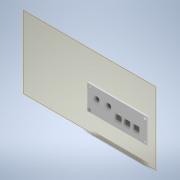
# Autodesk Inventor part: InterfacePlate
Saved by Autodesk Inventor 2022.2 (Build 262287000, 287)
## iProperties
Created: 2022-01-15
Part Number: InterfacePlate
Material: Generic
Document SubType Name: Modeling
Designer: siwat
Density: 1 g/cm^3
Appearance: Default
Author: siwat
Autodesk Inventor part; units mm, degrees
ref_plane "YZ Plane" through (0, 0, 0) normal (1, 0, 0) x (0, 1, 0)
ref_plane "XZ Plane" through (0, 0, 0) normal (0, 1, 0) x (-1, 0, 0)
ref_plane "XY Plane" through (0, 0, 0) normal (0, 0, 1) x (1, 0, 0)
ref_plane "Work Plane1" through (0, 0, 0) normal (0, 0, 1) x (1, 0, 0)
sketch "Sketch1" plane through (0, 0, 0) normal (0, 0, 1) x (1, 0, 0)
  line L0 (67.7271, 45.3897) -> (135.6749, 45.3897)
  line L1 (135.6749, 45.3897) -> (135.6749, 17.2701)
  line L2 (135.6749, 17.2701) -> (67.7271, 17.2701)
  line L3 (67.7271, 17.2701) -> (67.7271, 45.3897)
  circle A0 centre (70.3236, 42.7621) radius 1.5
  circle A1 centre (70.2655, 19.7679) radius 1.5
  circle A2 centre (132.8977, 19.6632) radius 1.5
  circle A3 centre (132.9442, 42.6673) radius 1.5
  point P0 (0, 0)
  dimension "d0" = 3
  dimension "d1" = 3
  dimension "d2" = 3
  dimension "d3" = 3
  constraints: 8 end point, 4 centre point, 2 parallel, 1 horizontal, 1 perpendicular
  measures "d0" diameter of A0
  measures "d1" diameter of A1
  measures "d2" diameter of A2
  measures "d3" diameter of A3
extrude "Extrusion1" add sketch "Sketch1" along normal blind 2
sketch "Sketch2" plane through (0, 0, 0) normal (0, 0, -1) x (-1, 0, 0)
  line L0 (-130.1897, 21.9638) -> (-72.4709, 21.9638)
  line L1 (-72.4709, 21.9638) -> (-72.4709, 40.332)
  line L2 (-72.4709, 40.332) -> (-130.1897, 40.332)
  line L3 (-130.1897, 40.332) -> (-130.1897, 21.9638)
  point P0 (0, 0)
  constraints: 8 end point, 2 parallel, 1 horizontal, 1 perpendicular
extrude "Extrusion2" add sketch "Sketch2" along normal blind 3
sketch "Sketch3" plane through (0, 0, -3) normal (0, 0, -1) x (-1, 0, 0)
  circle A0 centre (-123.1484, 27.6797) radius 2
  line L0 (-121.6186, 32.121) -> (-111.2555, 32.121)
  circle A1 centre (-113.1484, 27.6797) radius 2
  circle A2 centre (-103.1484, 27.6797) radius 2
  circle A3 centre (-91.5974, 33.7589) radius 2.65
  circle A4 centre (-78.3445, 33.7589) radius 2.65
  point P0 (0, 0)
  dimension "d8" = 4
  dimension "d11" = 10
  dimension "d16" = 5.3
  dimension "d17" = 5.3
  constraints: 5 centre point, 2 end point, 2 horizontal, 4 other
  measures "d8" diameter of A0
  measures "d11" distance of A0.centre A1.centre
  measures "d16" diameter of A3
  measures "d17" diameter of A4
extrude "Extrusion3" cut sketch "Sketch3" against normal up to surface (5 mm away)
sketch "Sketch5" plane through (0, 0, 2) normal (0, 0, 1) x (1, 0, 0)
  circle A0 centre (78.3445, 33.7589) radius 2.65 projected
  circle A1 centre (78.3445, 33.7589) radius 3.5
  circle A2 centre (91.5974, 33.7589) radius 2.65 projected
  circle A3 centre (91.5974, 33.7589) radius 3.5
  point P0 (0, 0)
  dimension "d22" = 7
  dimension "d23" = 7
  constraints: 2 centre point, 2 coincident
  measures "d22" diameter of A1
  measures "d23" diameter of A3
extrude "Extrusion5" cut sketch "Sketch5" against normal blind 0.5
sketch "Sketch6" plane through (0, 0, 2) normal (0, 0, 1) x (1, 0, 0)
  line L0 (99.7984, 31.0297) -> (106.4984, 31.0297)
  line L1 (106.4984, 31.0297) -> (106.4984, 24.3297)
  line L2 (106.4984, 24.3297) -> (99.7984, 24.3297)
  line L3 (99.7984, 24.3297) -> (99.7984, 31.0297)
  circle A0 centre (103.1484, 27.6797) radius 2 projected
  line L4 (109.7984, 31.0297) -> (116.4984, 31.0297)
  line L5 (116.4984, 31.0297) -> (116.4984, 24.3297)
  line L6 (116.4984, 24.3297) -> (109.7984, 24.3297)
  line L7 (109.7984, 24.3297) -> (109.7984, 31.0297)
  line L8 (119.7984, 31.0297) -> (126.4984, 31.0297)
  line L9 (126.4984, 31.0297) -> (126.4984, 24.3297)
  line L10 (126.4984, 24.3297) -> (119.7984, 24.3297)
  line L11 (119.7984, 24.3297) -> (119.7984, 31.0297)
  circle A1 centre (113.1484, 27.6797) radius 2 projected
  circle A2 centre (123.1484, 27.6797) radius 2 projected
  point P0 (0, 0)
  dimension "d26" = 6.7
  dimension "d27" = 6.7
  dimension "d28" = 3.35
  dimension "d29" = 3.35
  dimension "d30" = 6.7
  dimension "d31" = 6.7
  dimension "d32" = 6.7
  dimension "d33" = 6.7
  dimension "d34" = 3.35
  dimension "d35" = 3.35
  dimension "d36" = 3.35
  dimension "d37" = 3.35
  constraints: 24 end point, 6 parallel, 3 horizontal, 3 perpendicular
  measures "d26" distance of L1.end L2.end
  measures "d27" distance of L0.end L1.end
  measures "d28" distance from line of A0.centre L1
  measures "d29" distance from line of A0.centre L2
  measures "d30" distance of L5.end L6.end
  measures "d31" distance of L4.end L5.end
  measures "d32" distance of L9.end L10.end
  measures "d33" distance of L8.end L9.end
  measures "d34" distance from line of A1.centre L4
  measures "d35" distance from line of A2.centre L8
  measures "d36" distance from line of L5 A1.centre
  measures "d37" distance from line of L9 A2.centre
extrude "Extrusion6" cut sketch "Sketch6" against normal blind 3.5
equation "\"d28\" = 0.5 * d26"
equation "\"d29\" = 0.5 * d27"
equation "\"d34\" = 0.5 * d31"
equation "\"d35\" = 0.5 * d33"
equation "\"d36\" = 0.5 * d30"
equation "\"d37\" = 0.5 * d32"
body "Solid1"
